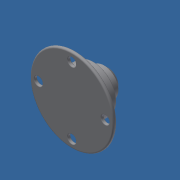
# Autodesk Inventor part: Podstawa
Saved by Autodesk Inventor 2014 SP1 (Build 180222100, 222)
## iProperties
Created: 2014-09-01
Part Number: Podstawa
Material: Ogólny
Document SubType Name: Modeling
Designer: Marcin
Density: 1 g/cm^3
Appearance: Domyślna
Author: Marcin
Autodesk Inventor part; units mm, degrees
ref_plane "YZ Plane" through (0, 0, 0) normal (1, 0, 0) x (0, 1, 0)
ref_plane "XZ Plane" through (0, 0, 0) normal (0, 1, 0) x (-1, 0, 0)
ref_plane "XY Plane" through (0, 0, 0) normal (0, 0, 1) x (1, 0, 0)
sketch "Szkic1" plane through (0, 0, 0) normal (0, 1, 0) x (-1, 0, 0)
  circle A0 centre (0, 0) radius 14.5
  circle A1 centre (0, -11.6) radius 1.4
  line L0 (0, -14.5) -> (0, 14.5)
  line L1 (14.5, 0) -> (-14.5, 0)
  circle A2 centre (-11.6, 0) radius 1.4
  circle A3 centre (0, 11.6) radius 1.4
  circle A4 centre (11.6, 0) radius 1.4
  dimension "podstawa" = 29
  dimension "d1" = 1.5
  dimension "d2" = 2.8
  dimension "d3" = 29
  dimension "d4" = 29
  dimension "d5" = 2.8
  dimension "d6" = 2.9
  constraints: 5 centre point, 4 end point, 4 point on circle, 2 point on line, 2 symmetric about line, 1 coincident, 1 perpendicular, 1 vertical, 2 other
  measures "podstawa" diameter of A0
  measures "d2" diameter of A1
  measures "d3" distance of L1.end L1.start
  measures "d4" distance of L0.start L0.end
  measures "d5" diameter of A2
  measures "d6" distance of A2.centre L1.end
extrude "Wyciągnięcie proste1" add sketch "Szkic1" along normal blind 1.2
sketch "Szkic2" plane through (0, 0, 0) normal (0, -1, 0) x (1, 0, 0)
  circle A0 centre (0, 11.6) radius 1.4 projected
  circle A1 centre (11.6, 0) radius 1.4 projected
  circle A2 centre (0, -11.6) radius 1.4 projected
  circle A3 centre (-11.6, 0) radius 1.4 projected
hole "Otwór1" at (0, 0, 11.6) at (11.6, 0, 0) at (-11.6, 0, 0) at (0, 0, -11.6) direction (0, 1, 0) diameter 2.8 end through all
fillet "Zaokrąglenie1" radius 0.5 4 edges at (0, 1.2, -10.2) (-11.6, 1.2, 1.4) (0, 1.2, 13) (11.6, 1.2, 1.4)
fillet "Zaokrąglenie2" radius 0.25 4 edges at (11.6, 0, 1.4) (0, 0, -10.2) (-11.6, 0, 1.4) (0, 0, 13)
fillet "Zaokrąglenie3" radius 0.5 2 edges at (0, 1.2, 14.5) (0, 0, 14.5)
sketch "Szkic3" plane through (0, 1.2, 0) normal (0, 1, 0) x (1, 0, 0)
  circle A0 centre (0, 0) radius 14 projected
  circle A1 centre (0, 0) radius 8
  dimension "d19" = 16
  constraints: 1 centre point, 1 coincident
  measures "d19" diameter of A1
extrude "Wyciągnięcie proste2" add sketch "Szkic3" along normal blind 6.5 contours A1
fillet "Zaokrąglenie4" radius 2 1 edges at (-8, 1.2, 0)
sketch "Szkic4" plane through (0, 7.7, 0) normal (0, 1, 0) x (1, 0, 0)
  circle A0 centre (0, 0) radius 8 projected
  circle A1 centre (0, 0) radius 5
  dimension "d23" = 10
  constraints: 1 centre point, 1 coincident
  measures "d23" diameter of A1
extrude "Wyciągnięcie proste3" add sketch "Szkic4" along normal blind 5 contours A1
chamfer "Faza1" distance 1.5 angle 45 1 edges at (-5, 12.7, 0)
fillet "Zaokrąglenie5" radius 0.5 2 edges at (-8, 7.7, 0) (-5, 7.7, 0)
equation "\"d3\" = podstawa"
equation "\"d4\" = podstawa"
equation "\"d5\" = d2"
equation "\"d6\" = d1 + 0.5 * d2"
equation "\"d9\" = d2"
